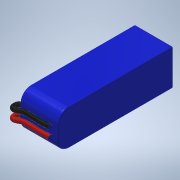
# Autodesk Inventor part: Battery4S
Saved by Autodesk Inventor 2020.2 (Build 242310000, 310)
## iProperties
Created: 2012-08-01
Part Number: Battery4S
Material: ABS Plastic
Document SubType Name: Modeling
Designer: rYan
Mass: 97.8232 g
Surface Area: 148.018 cm^2
Volume: 92.286 cm^3
Density: 1.06 g/cm^3
Description: TP1300-4SPR45
Vendor: Thunder Power
Appearance: Blue - Wall Paint - Glossy
Author: rYan
Autodesk Inventor part; units mm, degrees
ref_plane "YZ Plane" through (0, 0, 0) normal (1, 0, 0) x (0, 1, 0)
ref_plane "XZ Plane" through (0, 0, 0) normal (0, 1, 0) x (-1, 0, 0)
sketch "Skizze1" plane through (0, 0, 0) normal (0, 0, 1) x (1, 0, 0)
  line L0 (-17.5, 52.5) -> (17.5, 52.5)
  line L1 (17.5, 52.5) -> (17.5, -52.5)
  line L2 (17.5, -52.5) -> (-17.5, -52.5)
  line L3 (-17.5, -52.5) -> (-17.5, 52.5)
  line L4 (0, 73.5) -> (0, -73.5) projected
  line L5 (-24.5, 0) -> (24.5, 0) projected
  point P0 (0, 0)
  dimension "d0" = 35
  dimension "d2" = 105
  constraints: 8 end point, 2 parallel, 1 horizontal, 1 perpendicular, 2 other
  measures "d0" distance of L0.start L0.end
  measures "d2" distance of L0.end L1.end
extrude "Extrusion1" add sketch "Skizze1" along normal mid plane 33
fillet "Rundung1" radius 10 2 edges at (0, -52.5, -16.5) (0, -52.5, 16.5)
ref_plane "Arbeitsebene4" through (0, 0, 4) normal (0, 0, 1) x (1, 0, 0)
fillet "Rundung2" radius 1 14 edges at (0, 52.5, 16.5) (0, 52.5, -16.5) (-17.5, -49.5711, -13.5711) (-17.5, -52.5, 0) (-17.5, -49.5711, 13.5711) (-17.5, 5, 16.5) (-17.5, 5, -16.5) (17.5, -49.5711, -13.5711) (17.5, -52.5, 0) (17.5, -49.5711, 13.5711) (17.5, 5, 16.5) (17.5, 5, -16.5) (-17.5, 52.5, 0) (17.5, 52.5, 0)
sketch "Skizze10" plane through (-17.5, -42.5, -15.5) normal (-1, 0, 0) x (0, 0, 1)
  line L0 (19.5, -10.2235) -> (19.5, -8) projected
  circle A0 centre (19.5, -8) radius 2
  point P0 (15.5, 42.5)
  dimension "d42" = 4
  constraints: 1 centre point, 1 coincident
  measures "d42" diameter of A0
sketch "Skizze9" plane through (0, 0, 4) normal (0, 0, 1) x (1, 0, 0)
  arc A0 (-17.5, -50.5) -> (-20.3978, -52.7235) centre (-17.5, -53.5) ccw
  line L0 (-17.5, -53.5) -> (-20.3978, -52.7235) construction
  line L1 (-17.5, -53.5) -> (-17.5, -50.5) construction
  line L2 (16.5, -52.5) -> (-16.5, -52.5) projected
  line L3 (-17.5, -51.5) -> (-17.5, -42.5) projected
  arc A1 (-20.3978, -52.7235) -> (-20.398, -55.6026) centre (-15.0237, -54.1635) ccw
  arc A2 (-20.398, -55.6026) -> (-17.5001, -57.3753) centre (-18.0169, -54.965) ccw
  arc A3 (-17.5001, -57.3753) -> (-15.0238, -56.4892) centre (-19.5876, -47.6385) ccw
  arc A4 (-15.0238, -56.4892) -> (-13.5001, -55.603) centre (-22.9975, -41.0257) ccw
  arc A5 (-11.5001, -54.965) -> (-13.5001, -55.603) centre (-11.3414, -58.9164) ccw
  arc A6 (-1.5001, -55.1489) -> (-11.5001, -54.965) centre (-8.069, -140.3838) ccw
  arc A7 (-1.5001, -55.1489) -> (8.0613, -55.1489) centre (3.2806, 6.8844) ccw
  arc A8 (13.0425, -55.3328) -> (8.0613, -55.1489) centre (9.7474, -77.0264) ccw
  point P0 (-0.5, 0)
  dimension "d38" = 75
  dimension "d40" = 3
  dimension "d43" = 1
  dimension "d46" = 21.9424
  dimension "d47" = 62.2172
  dimension "d48" = 85.4877
  dimension "d49" = 3.9546
  dimension "d50" = 5.5637
  dimension "d51" = 2.465
  dimension "d52" = 9.958
  dimension "d53" = 17.3983
  dimension "d54" = 2.8328
  dimension "d55" = 30.5425
  dimension "d56" = 24.5264
  dimension "d57" = 2.6489
  dimension "d58" = 52.5
  dimension "d59" = 17
  dimension "d60" = 2.6489
  dimension "d61" = 6.4164
  dimension "d62" = 3.103
  constraints: 18 point on circle, 9 centre point, 9 tangent, 4 end point, 2 point on line
  measures "d38" angle of L1 L0
  measures "d40" radius of A0
  measures "d43" distance from line of L0.start L2
  measures "d46" radius of A8
  measures "d47" radius of A7
  measures "d48" radius of A6
  measures "d49" radius of A5
  measures "d50" radius of A1
  measures "d51" radius of A2
  measures "d52" radius of A3
  measures "d53" radius of A4
  measures "d54" distance from line of A8.start L2
  measures "d55" distance from line of A8.start L3
  measures "d56" distance from line of A8.centre L2
  measures "d57" distance from line of A7.end L2
  measures "d58" distance from line of point (-0.5, 0) L2
  measures "d59" distance from line of point (-0.5, 0) L3
  measures "d60" distance from line of A6.start L2
  measures "d61" distance from line of A5.centre L2
  measures "d62" distance from line of A4.end L2
sweep "Sweeping4" add profiles "Skizze10" path "Skizze9" path curves A0 A1 A2 A3 A4 A5 A6 A7 A8
mirror "Spiegeln3" about plane through (0, 0, 0) normal (0, 0, 1) of "Sweeping4"
